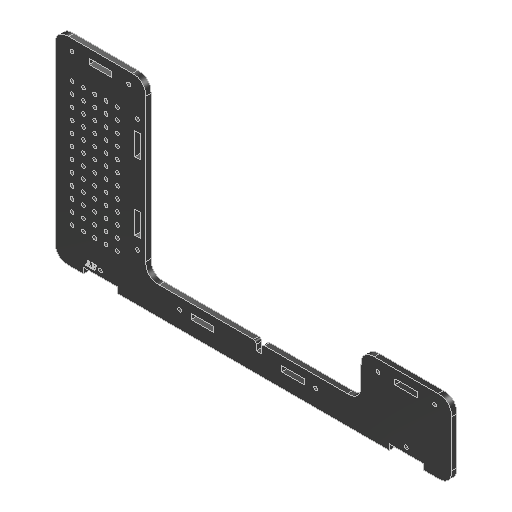
# Autodesk Inventor part: Mounting Side Wall
Saved by Autodesk Inventor 2025 (Build 290162000, 162)
## iProperties
Created: 2024-06-07
Part Number: Mounting Side Wall
Material: Polycarbonate, Clear
Document SubType Name: Modeling
Designer: AlexForbes
Density: 1.2 g/cm^3
Appearance: Glossy - Black
Author: AlexForbes
Autodesk Inventor part; units mm, degrees
ref_plane "YZ Plane" through (0, 0, 0) normal (1, 0, 0) x (0, 1, 0)
ref_plane "XZ Plane" through (0, 0, 0) normal (0, 1, 0) x (-1, 0, 0)
ref_plane "XY Plane" through (0, 0, 0) normal (0, 0, 1) x (1, 0, 0)
sketch "Sketch1" plane through (0, 0, 0) normal (0, 0, 1) x (1, 0, 0)
  line L0 (101.6, 31.75) -> (101.6, 222.25)
  line L1 (101.6, 222.25) -> (0, 222.25)
  line L2 (0, 222.25) -> (0, 0)
  line L3 (342.9, 31.75) -> (101.6, 31.75)
  line L4 (0, 0) -> (444.5, 0)
  line L5 (342.9, 31.75) -> (342.9, 82.55)
  line L6 (342.9, 82.55) -> (444.5, 82.55)
  line L7 (444.5, 0) -> (444.5, 82.55)
  dimension "d2" = 222.25
  dimension "d3" = 101.6
  dimension "d4" = 241.3
  dimension "d111" = 31.75
  dimension "d112" = 82.55
  constraints: 16 end point, 4 horizontal, 2 parallel, 2 vertical
  measures "d2" distance of L1.end L2.end
  measures "d3" distance of L0.end L1.end
  measures "d4" distance between parallel lines of L5 L0
  measures "d111" distance between parallel lines of L4 L3
  measures "d112" distance between parallel lines of L4 L6
extrude "Extrusion1" add sketch "Sketch1" along normal blind 6
sketch "Sketch2" plane through (0, 0, 6) normal (0, 0, 1) x (1, 0, 0)
  line L0 (38.1, 212.55) -> (63.5, 212.55)
  line L1 (63.5, 212.55) -> (63.5, 206.55)
  line L2 (63.5, 206.55) -> (38.1, 206.55)
  line L3 (38.1, 206.55) -> (38.1, 212.55)
  line L4 (89.25, 167.9) -> (95.25, 167.9)
  line L5 (95.25, 167.9) -> (95.25, 142.5)
  line L6 (95.25, 142.5) -> (89.25, 142.5)
  line L7 (89.25, 142.5) -> (89.25, 167.9)
  line L8 (89.25, 91.7) -> (95.25, 91.7)
  line L9 (95.25, 91.7) -> (95.25, 66.3)
  line L10 (95.25, 66.3) -> (89.25, 66.3)
  line L11 (89.25, 66.3) -> (89.25, 91.7)
  line L12 (152.4, 22.05) -> (177.8, 22.05)
  line L13 (177.8, 22.05) -> (177.8, 16.05)
  line L14 (177.8, 16.05) -> (152.4, 16.05)
  line L15 (152.4, 16.05) -> (152.4, 22.05)
  line L16 (254, 22.05) -> (279.4, 22.05)
  line L17 (279.4, 22.05) -> (279.4, 16.05)
  line L18 (279.4, 16.05) -> (254, 16.05)
  line L19 (254, 16.05) -> (254, 22.05)
  line L20 (406.4, 72.85) -> (381, 72.85)
  line L21 (381, 72.85) -> (381, 66.85)
  line L22 (381, 66.85) -> (406.4, 66.85)
  line L23 (406.4, 66.85) -> (406.4, 72.85)
  line L24 (92.25, 142.5) -> (92.25, 91.7) construction
  line L25 (177.8, 19.05) -> (254, 19.05) construction
  line L26 (393.7, 66.85) -> (393.7, 72.85) construction
  line L27 (50.8, 206.55) -> (50.8, 212.55) construction
  line L28 (0, 222.25) -> (0, 0) projected
  line L29 (0, 0) -> (444.5, 0) projected
  point P0 (89.25, 79)
  point P1 (89.25, 155.2)
  point P2 (215.9, 19.05)
  point P3 (50.8, 209.55)
  point P4 (92.25, 117.1)
  dimension "d7" = 6
  dimension "d50" = 76.2
  dimension "d76" = 139.7
  dimension "d79" = 25.4
  dimension "d80" = 31.75
  dimension "d91" = 190.5
  dimension "d93" = 50.8
  dimension "d94" = 165.1
  dimension "d95" = 342.9
  dimension "d97" = 209.55
  dimension "d99" = 89.45
  dimension "d100" = 76.2
  constraints: 56 end point, 13 midpoint, 9 equal length, 9 parallel, 6 horizontal, 5 vertical, 4 perpendicular, 3 point on line
  measures "d7" distance of L2.end L0.start
  measures "d50" distance of L25.start L25.end
  measures "d76" distance between parallel lines of L0 L20
  measures "d79" distance of L0.start L0.end
  measures "d80" distance between parallel lines of L5 L1
  measures "d91" distance between parallel lines of L12 L0
  measures "d93" distance between parallel lines of L28 L27
  measures "d94" distance from line of point (215.9, 19.05) L27
  measures "d95" distance between parallel lines of L27 L26
  measures "d97" distance from line of L29 point (50.8, 209.55)
  measures "d99" distance from line of point (92.25, 117.1) L2
  measures "d100" distance of point (89.25, 79) point (89.25, 155.2)
extrude "Extrusion2" cut sketch "Sketch2" against normal blind 6
sketch "Sketch3" plane through (0, 0, 6) normal (0, 0, 1) x (1, 0, 0)
  line L0 (31.75, 0) -> (69.85, 0)
  line L1 (69.85, 0) -> (69.85, 6.35)
  line L2 (69.85, 6.35) -> (31.75, 6.35)
  line L3 (31.75, 6.35) -> (31.75, 0)
  line L4 (374.65, 0) -> (412.75, 0)
  line L5 (412.75, 0) -> (412.75, 6.35)
  line L6 (412.75, 6.35) -> (374.65, 6.35)
  line L7 (374.65, 6.35) -> (374.65, 0)
  line L8 (50.8, 12.7) -> (50.8, 6.35) construction
  line L9 (393.7, 12.7) -> (393.7, 6.35) construction
  line L10 (101.6, 222.25) -> (0, 222.25) projected
  line L11 (444.5, 82.55) -> (342.9, 82.55) projected
  line L12 (0, 0) -> (444.5, 0) construction
  line L13 (196.85, 0) -> (234.95, 0) construction
  line L14 (234.95, 0) -> (234.95, 6.35) construction
  line L15 (234.95, 6.35) -> (196.85, 6.35) construction
  line L16 (196.85, 6.35) -> (196.85, 0) construction
  line L17 (215.9, 6.35) -> (215.9, 12.7) construction
  line L18 (342.9, 31.75) -> (101.6, 31.75) construction
  line L19 (177.8, 16.05) -> (177.8, 22.05) projected
  line L20 (177.8, 19.05) -> (254, 19.05) construction
  line L21 (254, 22.05) -> (254, 16.05) construction
  point P0 (50.8, 0)
  point P1 (50.8, 222.25)
  point P2 (393.7, 0)
  point P3 (393.7, 82.55)
  point P4 (215.9, 19.05)
  dimension "d11" = 6.35
  dimension "d12" = 38.1
  dimension "d98" = 12.7
  constraints: 32 end point, 10 midpoint, 6 parallel, 4 equal length, 4 point on line, 3 horizontal, 3 perpendicular, 3 vertical, 3 vertical alignment, 1 horizontal alignment
  measures "d11" distance of L0.end L1.end
  measures "d12" distance of L1.end L2.end
  measures "d98" distance from line of L12 L8.start
sketch "Sketch5" plane through (0, 0, 6) normal (0, 0, 1) x (1, 0, 0)
  line L0 (381, 66.85) -> (381, 72.85) projected
  line L1 (406.4, 72.85) -> (406.4, 66.85) projected
  line L2 (279.4, 22.05) -> (279.4, 16.05) projected
  line L3 (152.4, 16.05) -> (152.4, 22.05) projected
  line L4 (63.5, 212.55) -> (63.5, 206.55) projected
  line L5 (38.1, 206.55) -> (38.1, 212.55) projected
  line L6 (89.25, 167.9) -> (95.25, 167.9) projected
  line L7 (89.25, 91.7) -> (95.25, 91.7) projected
  line L8 (19.05, 209.55) -> (82.55, 209.55) construction
  line L9 (38.1, 212.55) -> (63.5, 212.55) projected
  line L10 (361.95, 69.85) -> (425.45, 69.85) construction
  line L11 (92.25, 53.6) -> (92.25, 180.6) construction
  line L12 (139.7, 19.05) -> (292.1, 19.05) construction
  line L13 (89.25, 142.5) -> (95.25, 142.5) projected
  line L14 (95.25, 142.5) -> (95.25, 91.7) construction
  line L15 (95.25, 91.7) -> (95.25, 66.3) construction
  line L16 (95.25, 66.3) -> (89.25, 66.3) construction
  line L17 (89.25, 66.3) -> (89.25, 91.7) construction
  line L18 (89.25, 91.7) -> (95.25, 91.7) construction
  line L19 (381, 72.85) -> (406.4, 72.85) construction
  line L20 (406.4, 72.85) -> (406.4, 66.85) construction
  line L21 (406.4, 66.85) -> (381, 66.85) construction
  line L22 (381, 66.85) -> (381, 72.85) construction
  line L23 (95.25, 167.9) -> (95.25, 142.5) construction
  line L24 (95.25, 142.5) -> (89.25, 142.5) construction
  line L25 (89.25, 142.5) -> (89.25, 167.9) construction
  line L26 (89.25, 167.9) -> (95.25, 167.9) construction
  line L27 (177.8, 22.05) -> (177.8, 16.05) construction
  line L28 (177.8, 16.05) -> (152.4, 16.05) construction
  line L29 (152.4, 16.05) -> (152.4, 22.05) construction
  line L30 (152.4, 22.05) -> (177.8, 22.05) construction
  line L31 (279.4, 22.05) -> (279.4, 16.05) construction
  line L32 (279.4, 16.05) -> (254, 16.05) construction
  line L33 (254, 16.05) -> (254, 22.05) construction
  line L34 (254, 22.05) -> (279.4, 22.05) construction
  line L35 (63.5, 212.55) -> (63.5, 206.55) construction
  line L36 (63.5, 206.55) -> (38.1, 206.55) construction
  line L37 (38.1, 206.55) -> (38.1, 212.55) construction
  line L38 (101.6, 222.25) -> (0, 222.25) construction
  line L39 (0, 222.25) -> (0, 0) construction
  line L40 (0, 0) -> (444.5, 0) construction
  line L41 (444.5, 0) -> (444.5, 82.55) construction
  line L42 (444.5, 82.55) -> (342.9, 82.55) construction
  line L43 (342.9, 82.55) -> (342.9, 31.75) construction
  line L44 (342.9, 31.75) -> (101.6, 31.75) construction
  line L45 (101.6, 31.75) -> (101.6, 222.25) construction
  line L46 (177.8, 19.05) -> (254, 19.05) construction
  line L47 (38.1, 212.55) -> (63.5, 212.55) projected
  point P0 (381, 69.85)
  point P1 (406.4, 69.85)
  point P2 (279.4, 19.05)
  point P3 (152.4, 19.05)
  point P4 (92.25, 167.9)
  point P5 (92.25, 91.7)
  point P6 (50.8, 209.55)
  point P7 (50.8, 212.55)
  point P8 (393.7, 69.85)
  point P9 (92.25, 117.1)
  point P10 (95.25, 117.1)
  point P11 (393.7, 72.85)
  point P12 (38.1, 209.55)
  point P13 (215.9, 19.05)
  dimension "d47" = 63.5
  dimension "d52" = 127
  dimension "d53" = 152.4
  constraints: 17 midpoint, 12 end point, 6 horizontal alignment, 4 vertical alignment, 3 horizontal, 1 parallel, 1 perpendicular, 1 point on line, 1 vertical
  measures "d47" distance of L8.end L8.start
  measures "d52" distance of L11.start L11.end
  measures "d53" distance of L12.start L12.end
hole "Hole3" at (19.05, 209.55, 6) at (82.55, 209.55, 6) at (92.25, 180.6, 6) at (92.25, 53.6, 6) at (139.7, 19.05, 6) at (292.1, 19.05, 6) at (361.95, 69.85, 6) at (425.45, 69.85, 6) direction (0, 0, -1) diameter 4.25 end through all
sketch "Sketch4" plane through (0, 0, 6) normal (0, 0, 1) x (1, 0, 0)
  line L0 (101.6, 222.25) -> (0, 222.25) projected
  line L1 (0, 222.25) -> (0, 0) projected
  line L2 (0, 0) -> (444.5, 0) projected
  point P0 (19.05, 180.8)
  dimension "d25" = 19.05
  dimension "d92" = 180.8
  measures "d25" distance from line of point (19.05, 180.8) L1
  measures "d92" distance from line of L2 point (19.05, 180.8)
hole "Hole2" at (19.05, 180.8, 6) direction (0, 0, -1) diameter 4.25 end through all
pattern_linear "Rectangular Pattern1" count 12 spacing 12.7 along (0, -1, 0) count 5 spacing 12.7 along (1, 0, 0) of "Hole2"
extrude "Extrusion3" cut sketch "Sketch3" against normal blind 6
hole "Hole1" at (50.8, 12.7, 6) at (393.7, 12.7, 6) direction (0, 0, -1) diameter 4.25 end through all
sketch "Sketch6" plane through (0, 0, 6) normal (0, 0, 1) x (1, 0, 0)
  line L0 (342.9, 31.75) -> (101.6, 31.75) construction
  line L1 (225.6, 31.75) -> (231.6, 31.75)
  line L2 (231.6, 31.75) -> (231.6, 22.225)
  line L3 (231.6, 22.225) -> (225.6, 22.225)
  line L4 (225.6, 22.225) -> (225.6, 31.75)
  line L5 (0, 222.25) -> (0, 0) construction
  point P0 (228.6, 31.75)
  dimension "d103" = 6
  dimension "d104" = 9.525
  dimension "d105" = 228.6
  constraints: 8 end point, 2 parallel, 1 horizontal, 1 midpoint, 1 perpendicular, 1 point on line
  measures "d103" distance between parallel lines of L2 L4
  measures "d104" distance between parallel lines of L0 L3
  measures "d105" distance from line of L5 point (228.6, 31.75)
extrude "Extrusion4" cut sketch "Sketch6" against normal through all
fillet "Fillet1" radius 15 8 edges at (101.6, 222.25, 3) (0, 222.25, 3) (101.6, 31.75, 3) (444.5, 82.55, 3) (342.9, 82.55, 3) (342.9, 31.75, 3) (0, 0, 3) (444.5, 0, 3) curvature continuous yes
fillet "Fillet2" radius 3.175 2 edges at (225.6, 31.75, 3) (231.6, 31.75, 3)
sketch "Sketch7" plane through (0, 0, 6) normal (0, 0, 1) x (1, 0, 0)
  line L0 (31.75, 19.05) -> (48.675, 19.05) construction
  line L1 (48.675, 19.05) -> (48.675, 6.35) construction
  line L2 (48.675, 6.35) -> (31.75, 6.35) construction
  line L3 (31.75, 6.35) -> (31.75, 19.05) construction
  circle A0 centre (50.8, 12.7) radius 2.125 construction
  line L4 (40.8323, 9.6105) -> (37.5135, 9.6105)
  line L5 (37.5135, 9.6105) -> (37.5135, 9.9473)
  spline S0 degree 2 poles (37.5135, 9.9473) (37.7477, 9.9668) (38.3725, 10.0986) (38.3725, 10.1962) knots 0 0 0 1 2 2 2
  spline S1 degree 2 poles (38.3725, 10.1962) (38.3725, 10.2304) (38.3578, 10.3182) (38.3285, 10.3914) knots 0 0 0 1 2 2 2
  line L6 (38.3285, 10.3914) -> (37.8112, 11.6506)
  line L7 (37.8112, 11.6506) -> (35.7076, 11.6506)
  spline S2 degree 2 poles (35.7076, 11.6506) (35.6344, 11.4749) (35.4587, 11.0015) (35.3952, 10.816) knots 0 0 0 1 2 2 2
  spline S3 degree 2 poles (35.3952, 10.816) (35.3123, 10.5769) (35.283, 10.3621) (35.283, 10.3182) knots 0 0 0 1 2 2 2
  spline S4 degree 2 poles (35.283, 10.3182) (35.283, 10.1816) (35.7027, 9.9912) (36.1859, 9.9473) knots 0 0 0 1 2 2 2
  line L8 (36.1859, 9.9473) -> (36.1859, 9.6105)
  line L9 (36.1859, 9.6105) -> (33.687, 9.6105)
  line L10 (33.687, 9.6105) -> (33.687, 9.9473)
  spline S5 degree 2 poles (33.687, 9.9473) (33.8285, 9.957) (34.1848, 10.0303) (34.2873, 10.0937) knots 0 0 0 1 2 2 2
  spline S6 degree 2 poles (34.2873, 10.0937) (34.463, 10.1962) (34.7071, 10.4988) (34.79, 10.7038) knots 0 0 0 1 2 2 2
  spline S7 degree 2 poles (34.79, 10.7038) (35.2879, 11.9093) (36.2884, 14.3302) (36.8936, 15.7895) knots 0 0 0 1 2 2 2
  line L11 (36.8936, 15.7895) -> (37.7526, 15.7895)
  spline S8 degree 2 poles (37.7526, 15.7895) (38.5921, 13.7201) (39.5438, 11.3188) (39.8806, 10.5281) knots 0 0 0 1 2 2 2
  spline S9 degree 2 poles (39.8806, 10.5281) (39.9343, 10.3963) (40.1051, 10.1864) (40.2662, 10.0937) knots 0 0 0 1 2 2 2
  spline S10 degree 2 poles (40.2662, 10.0937) (40.3882, 10.0254) (40.7055, 9.957) (40.8323, 9.9473) knots 0 0 0 1 2 2 2
  line L12 (40.8323, 9.9473) -> (40.8323, 9.6105)
  line L13 (37.6355, 12.0753) -> (36.7521, 14.2813)
  line L14 (36.7521, 14.2813) -> (35.8833, 12.0753)
  line L15 (35.8833, 12.0753) -> (37.6355, 12.0753)
  line L16 (46.3671, 14.0812) -> (46.0303, 14.0812)
  spline S11 degree 2 poles (46.0303, 14.0812) (45.9083, 14.4375) (45.2738, 15.2331) (44.9907, 15.2721) knots 0 0 0 1 2 2 2
  spline S12 degree 2 poles (44.9907, 15.2721) (44.8638, 15.2917) (44.4343, 15.3161) (44.2537, 15.3161) knots 0 0 0 1 2 2 2
  line L17 (44.2537, 15.3161) -> (43.3069, 15.3161)
  line L18 (43.3069, 15.3161) -> (43.3069, 12.9294)
  line L19 (43.3069, 12.9294) -> (43.9121, 12.9294)
  spline S13 degree 2 poles (43.9121, 12.9294) (44.1708, 12.9294) (44.5466, 13.0465) (44.693, 13.193) knots 0 0 0 1 2 2 2
  spline S14 degree 2 poles (44.693, 13.193) (44.8004, 13.3003) (45.0054, 13.803) (45.0249, 13.9836) knots 0 0 0 1 2 2 2
  line L20 (45.0249, 13.9836) -> (45.3519, 13.9836)
  line L21 (45.3519, 13.9836) -> (45.3519, 11.4213)
  line L22 (45.3519, 11.4213) -> (45.0249, 11.4213)
  spline S15 degree 2 poles (45.0249, 11.4213) (45.0054, 11.6165) (44.776, 12.168) (44.693, 12.2607) knots 0 0 0 1 2 2 2
  spline S16 degree 2 poles (44.693, 12.2607) (44.571, 12.3974) (44.1854, 12.5292) (43.9121, 12.5292) knots 0 0 0 1 2 2 2
  line L23 (43.9121, 12.5292) -> (43.3069, 12.5292)
  line L24 (43.3069, 12.5292) -> (43.3069, 10.5086)
  spline S17 degree 2 poles (43.3069, 10.5086) (43.3069, 10.3573) (43.424, 10.1376) (43.5851, 10.0693) knots 0 0 0 1 2 2 2
  spline S18 degree 2 poles (43.5851, 10.0693) (43.6827, 10.0303) (44.0146, 9.9668) (44.1756, 9.9473) knots 0 0 0 1 2 2 2
  line L25 (44.1756, 9.9473) -> (44.1756, 9.6105)
  line L26 (44.1756, 9.6105) -> (40.8909, 9.6105)
  line L27 (40.8909, 9.6105) -> (40.8909, 9.9473)
  spline S19 degree 2 poles (40.8909, 9.9473) (41.0178, 9.9619) (41.4278, 10.0059) (41.5108, 10.04) knots 0 0 0 1 2 2 2
  spline S20 degree 2 poles (41.5108, 10.04) (41.6621, 10.1035) (41.7841, 10.3182) (41.7841, 10.4842) knots 0 0 0 1 2 2 2
  line L28 (41.7841, 10.4842) -> (41.7841, 14.7792)
  spline S21 degree 2 poles (41.7841, 14.7792) (41.7841, 14.9256) (41.6767, 15.1452) (41.5108, 15.2184) knots 0 0 0 1 2 2 2
  spline S22 degree 2 poles (41.5108, 15.2184) (41.3887, 15.2721) (40.9934, 15.3551) (40.8909, 15.3697) knots 0 0 0 1 2 2 2
  line L29 (40.8909, 15.3697) -> (40.8909, 15.7065)
  line L30 (40.8909, 15.7065) -> (46.3671, 15.7065)
  line L31 (46.3671, 15.7065) -> (46.3671, 14.0812)
  point P0 (0, 0)
  point P1 (48.675, 12.7)
  constraints: 1 coincident, 1 horizontal alignment, 1 midpoint, 1 tangent, 1 vertical, 2 other
emboss "Emboss1" sketch "Sketch7" operation cut depth 2.54 direction (0, 0, -1)
body "Solid1"
